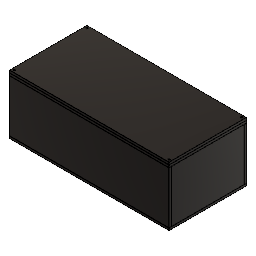
Battery Box ABS Panel v19 (Autodesk Fusion 360 design; units mm, degrees)
Autodesk Fusion 360 part; units mm, degrees
sketch "Sketch1" plane through (0, 0, 0) normal (0, 1, 0) x (1, 0, 0)
  line L0 (197.5, -96) -> (-197.5, -96)
  line L1 (-197.5, -96) -> (-197.5, 96)
  line L2 (-197.5, 96) -> (197.5, 96)
  line L3 (197.5, 96) -> (197.5, -96)
  line L4 (197.5, -96) -> (-197.5, 96) construction
  line L5 (-197.5, -96) -> (197.5, 96) construction
  line L6 (-197.5, 0) -> (197.5, 0) construction
  line L7 (0, 96) -> (0, -96) construction
  dimension "loa" = 395
  dimension "woa" = 192
  constraint horizontal L0
  constraint perpendicular L0 L1
  constraint parallel L0 L2
  constraint parallel L1 L3
  constraint coincident L4 origin
  constraint coincident L5 origin
  constraint midpoint L1 L6.start
  constraint midpoint L3 L6.end
  constraint midpoint L2 L7.start
  constraint midpoint L0 L7.end
  measures "loa" distance of L1.end L2.end
  measures "woa" distance of L0.end L1.end
extrude "Extrude1" add sketch "Sketch1" along normal blind 6 makes body 1
sketch "Sketch9" plane through (0, 6, 0) normal (0, 1, 0) x (-1, 0, 0)
  line L0 (-197.5, -96) -> (197.5, -96)
  line L1 (197.5, -96) -> (197.5, 96)
  line L2 (-197.5, 96) -> (-197.5, -96)
  circle A0 centre (191.5, -90) radius 3
  line L3 (195.85, -71) -> (195.85, -74.7217)
  arc A1 (190.1785, -83.3177) -> (195.85, -74.7217) centre (186.5, -74.7217) ccw
  line L4 (190.1785, -83.3177) -> (187.9545, -84.2694)
  arc A2 (187.9545, -84.2694) -> (185.4753, -86.7956) centre (189.7839, -88.5444) ccw
  line L5 (184.7768, -88.5165) -> (185.4753, -86.7956)
  arc A3 (176.1133, -94.35) -> (184.7768, -88.5165) centre (176.1133, -85) ccw
  line L6 (172.5, -94.35) -> (176.1133, -94.35)
  line L7 (172.5, -91.65) -> (176.1133, -91.65)
  arc A4 (176.1133, -91.65) -> (182.275, -87.501) centre (176.1133, -85) ccw
  line L8 (182.275, -87.501) -> (182.9735, -85.7802)
  arc A5 (186.8923, -81.7871) -> (182.9735, -85.7802) centre (189.7839, -88.5444) ccw
  line L9 (189.1162, -80.8354) -> (186.8923, -81.7871)
  arc A6 (189.1162, -80.8354) -> (193.15, -74.7217) centre (186.5, -74.7217) ccw
  line L10 (193.15, -71) -> (193.15, -74.7217)
  line L11 (197.5, 0.1916) -> (197.5, -96)
  line L12 (197.5, -96) -> (0, -96)
  line L13 (193.15, -71) -> (193.0809, 0.1873)
  line L14 (195.85, -71) -> (195.7809, 0.1899)
  line L15 (172.5, -94.35) -> (0, -94.35)
  line L16 (172.5, -91.65) -> (0, -91.65)
  line L17 (172.5, -90) -> (0, -90)
  line L18 (172.5, -90) -> (176.1133, -90)
  arc A7 (176.1133, -90) -> (180.7462, -86.8805) centre (176.1133, -85) ccw
  line L19 (180.7462, -86.8805) -> (181.4446, -85.1596)
  arc A8 (186.2431, -80.2702) -> (181.4446, -85.1596) centre (189.7839, -88.5444) ccw
  line L20 (188.4671, -79.3185) -> (186.2431, -80.2702)
  arc A9 (188.4671, -79.3185) -> (191.5, -74.7217) centre (186.5, -74.7217) ccw
  line L21 (191.5, -71.0008) -> (191.5, -74.7217)
  line L22 (191.5, -71.0008) -> (191.4309, 0.1857)
  line L23 (197.5, 0.1916) -> (191.4309, 0.1857)
  line L24 (0, -96) -> (0, -90)
  point P0 (191.5, -80.0006)
  point P1 (181.5, -80.0006)
  point P2 (181.5, -90.0006)
  point P3 (194.5, -80)
  point P4 (181.5, -93)
  dimension "d74" = 10
  dimension "d75" = 10
  dimension "d80" = 6
  dimension "d97" = 6
  dimension "d98" = 6
  dimension "d99" = -1.65
  constraint coincident L0.end L1.start
  constraint tangent L5 A3
  constraint tangent L4 A2
  constraint tangent A3 L6
  constraint tangent L3 A1
  constraint tangent A2 L5
  constraint tangent A1 L4
  constraint tangent A6 L10
  constraint tangent L9 A6
  constraint tangent A5 L9
  constraint tangent A4 L8
  constraint tangent L7 A4
  constraint tangent L8 A5
  constraint vertical L11
  constraint horizontal L12
  constraint perpendicular L22 L23
  constraint perpendicular L17 L24
  measures "d74" distance of P0 P1
  measures "d75" distance of P1 P2
  measures "d80" diameter of A0
  measures "d97" distance of A0.centre L12
  measures "d98" distance of A0.centre L11
sketch "Sketch2" plane through (0, 6, 0) normal (0, 1, 0) x (-1, 0, 0)
  line L0 (-181, 79.5) -> (181, 79.5)
  line L1 (181, 79.5) -> (181, -79.5)
  line L2 (181, -79.5) -> (-181, -79.5)
  line L3 (-181, -79.5) -> (-181, 79.5)
  line L4 (-181, 79.5) -> (181, -79.5) construction
  line L5 (181, 79.5) -> (-181, -79.5) construction
  line L6 (183, 81.5) -> (183, -81.5)
  line L7 (183, -81.5) -> (-183, -81.5)
  line L8 (-183, -81.5) -> (-183, 81.5)
  line L9 (-183, 81.5) -> (183, 81.5)
  line L10 (-197.5, -96) -> (197.5, -96)
  line L11 (197.5, -96) -> (197.5, 96)
  line L12 (197.5, 96) -> (-197.5, 96)
  line L13 (-197.5, 96) -> (-197.5, -96)
  dimension "d14" = 159
  dimension "d15" = 362
  dimension "d16" = -2
  constraint horizontal L0
  constraint perpendicular L0 L1
  constraint parallel L0 L2
  constraint parallel L1 L3
  constraint coincident L4 origin
  constraint coincident L5 origin
  measures "d14" distance of L0.end L1.end
  measures "d15" distance of L1.end L2.end
sketch "Sketch3" plane through (0, 6, 0) normal (0, 1, 0) x (-1, 0, 0)
  line L0 (-180, 78.5) -> (180, 78.5)
  line L1 (180, 78.5) -> (180, -78.5)
  line L2 (180, -78.5) -> (-180, -78.5)
  line L3 (-180, -78.5) -> (-180, 78.5)
  line L4 (-180, 78.5) -> (180, -78.5) construction
  line L5 (180, 78.5) -> (-180, -78.5) construction
  line L6 (-197.5, -96) -> (197.5, -96)
  line L7 (197.5, -96) -> (197.5, 96)
  line L8 (197.5, 96) -> (-197.5, 96)
  line L9 (-197.5, 96) -> (-197.5, -96)
  dimension "d19" = 360
  dimension "d20" = 157
  constraint horizontal L0
  constraint perpendicular L0 L1
  constraint parallel L0 L2
  constraint parallel L1 L3
  constraint coincident L4 origin
  constraint coincident L5 origin
  measures "d19" distance of L1.end L2.end
  measures "d20" distance of L0.end L1.end
extrude "Extrude4" add sketch "Sketch3" along normal blind 80 separate body contours L0 L1 L2 L3 makes body 2
sketch "Sketch4" plane through (0, 86, 0) normal (0, 1, 0) x (-1, 0, 0)
  line L0 (-180, -78.5) -> (180, -78.5)
  line L1 (180, -78.5) -> (180, 78.5)
  line L2 (180, 78.5) -> (-180, 78.5)
  line L3 (-180, 78.5) -> (-180, -78.5)
  line L4 (-42.5, 65) -> (42.5, 65)
  line L5 (42.5, 65) -> (42.5, -65)
  line L6 (42.5, -65) -> (-42.5, -65)
  line L7 (-42.5, -65) -> (-42.5, 65)
  line L8 (-42.5, 65) -> (42.5, -65) construction
  line L9 (42.5, 65) -> (-42.5, -65) construction
  dimension "d23" = 85
  dimension "d24" = 130
  constraint horizontal L4
  constraint perpendicular L4 L5
  constraint parallel L4 L6
  constraint parallel L5 L7
  constraint coincident L8 origin
  constraint coincident L9 origin
  measures "d23" distance of L5.end L6.end
  measures "d24" distance of L4.end L5.end
extrude "Extrude5" add sketch "Sketch4" along normal blind 36 separate body contours L4 L5 L6 L7 makes body 3
box "BoxPrimitive1" add length 6 width 395 height 129 placed x (0, 0, 1) y (1, 0, 0) z (0, 1, 0) at (-197.5, 6, -96) separate body makes body 4
mirror "Mirror3" about plane through (0, 0, 0) normal (0, 0, 1) of bodies 4 makes body 5
sketch "Sketch14" plane through (0, 6, 0) normal (0, 1, 0) x (-1, 0, 0)
  line L0 (-197.5, -96) -> (197.5, -96)
  line L1 (197.5, -96) -> (197.5, 96)
  line L2 (197.5, 96) -> (-197.5, 96)
  line L3 (-197.5, 96) -> (-197.5, -96)
  line L4 (197.5, 90) -> (-197.5, 90)
  line L5 (-197.5, -90) -> (197.5, -90)
  line L6 (197.5, 90) -> (191.5, 90)
  line L7 (191.5, 90) -> (191.5, -90)
  line L8 (191.5, -90) -> (197.5, -90)
  line L9 (197.5, -90) -> (197.5, 90)
  dimension "d118" = 6
  constraint horizontal L6
  constraint vertical L7
  constraint horizontal L8
  constraint vertical L9
  constraint coincident L4.start L6.start
  measures "d118" distance of L4.start L6.end
extrude "Extrude13" add sketch "Sketch14" along normal blind 129 separate body contours L1 L4 L5 L6 L7 L8 L9 makes body 6
mirror "Mirror4" about plane through (0, 0, 0) normal (1, 0, 0) of bodies 6 makes body 7
sketch "Sketch16" plane through (0, 135, 0) normal (0, 1, 0) x (-1, 0, 0)
  line L0 (197.5, -90) -> (-197.5, -90)
  line L1 (-197.5, -90) -> (-197.5, -96)
  line L2 (-197.5, -96) -> (197.5, -96)
  line L3 (197.5, -96) -> (197.5, -90)
  line L4 (197.5, -96) -> (0, -96)
  line L5 (197.5, 0.1916) -> (197.5, -96)
  line L6 (191.5, -71.0008) -> (191.4309, 0.1857)
  line L7 (172.5, -94.35) -> (0, -94.35)
  line L8 (172.5, -91.65) -> (0, -91.65)
  line L9 (172.5, -90) -> (0, -90)
  line L10 (172.5, -94.35) -> (176.1133, -94.35)
  arc A0 (176.1133, -94.35) -> (184.7768, -88.5165) centre (176.1133, -85) ccw
  circle A1 centre (191.5, -90) radius 3
  line L11 (184.7768, -88.5165) -> (185.4753, -86.7956)
  arc A2 (187.9545, -84.2694) -> (185.4753, -86.7956) centre (189.7839, -88.5444) ccw
  line L12 (190.1785, -83.3177) -> (187.9545, -84.2694)
  arc A3 (190.1785, -83.3177) -> (195.85, -74.7217) centre (186.5, -74.7217) ccw
  line L13 (195.85, -71) -> (195.85, -74.7217)
  line L14 (195.85, -71) -> (195.7809, 0.1899)
  line L15 (193.15, -71) -> (193.0809, 0.1873)
  line L16 (193.15, -71) -> (193.15, -74.7217)
  line L17 (191.5, -71.0008) -> (191.5, -74.7217)
  arc A4 (189.1162, -80.8354) -> (193.15, -74.7217) centre (186.5, -74.7217) ccw
  line L18 (189.1162, -80.8354) -> (186.8923, -81.7871)
  arc A5 (188.4671, -79.3185) -> (191.5, -74.7217) centre (186.5, -74.7217) ccw
  line L19 (188.4671, -79.3185) -> (186.2431, -80.2702)
  arc A6 (186.2431, -80.2702) -> (181.4446, -85.1596) centre (189.7839, -88.5444) ccw
  arc A7 (186.8923, -81.7871) -> (182.9735, -85.7802) centre (189.7839, -88.5444) ccw
  line L20 (182.275, -87.501) -> (182.9735, -85.7802)
  line L21 (180.7462, -86.8805) -> (181.4446, -85.1596)
  arc A8 (176.1133, -91.65) -> (182.275, -87.501) centre (176.1133, -85) ccw
  line L22 (172.5, -91.65) -> (176.1133, -91.65)
  line L23 (172.5, -90) -> (176.1133, -90)
  arc A9 (176.1133, -90) -> (180.7462, -86.8805) centre (176.1133, -85) ccw
  line L24 (197.5, 0.1916) -> (191.4309, 0.1857)
  line L25 (0, -96) -> (0, -90)
  constraint coincident L5.start L24.start
  constraint coincident L6.end L24.end
  constraint coincident L4.end L25.start
  constraint coincident L9.end L25.end
extrude "Extrude14" add sketch "Sketch16" along normal blind 6 separate body contours L0 L2 L3 L4 L5 L7 L10 A0 A1 L25 | L0 L5 A0 A1 L11 A2 L12 A3 L13 L14 L24 | L0 A0 L11 A2 L12 A3 L13 L14 L15 L16 A4 L18 A7 L20 A8 L24 | L0 L7 L8 L10 A0 A8 L22 L25 | L0 L6 L15 L16 L17 A4 L18 A5 L19 A6 A7 L20 L21 A8 A9 L24 | L0 L8 L9 A8 L22 L23 L25 makes body 8
sketch "Sketch17" plane through (0, 141, 0) normal (0, 1, 0) x (-1, 0, 0)
  circle A0 centre (191.5, -90) radius 3
  line L0 (197.5, 0.1916) -> (191.4309, 0.1857)
  line L1 (191.4309, 0.1857) -> (191.5, -71.0008)
  line L2 (191.5, -71.0008) -> (191.5, -74.7217)
  arc A1 (188.4671, -79.3185) -> (191.5, -74.7217) centre (186.5, -74.7217) ccw
  line L3 (188.4671, -79.3185) -> (186.2431, -80.2702)
  arc A2 (186.2431, -80.2702) -> (181.4446, -85.1596) centre (189.7839, -88.5444) ccw
  line L4 (181.4446, -85.1596) -> (180.7462, -86.8805)
  arc A3 (176.1133, -90) -> (180.7462, -86.8805) centre (176.1133, -85) ccw
  line L5 (176.1133, -90) -> (172.5, -90)
  line L6 (172.5, -90) -> (0, -90)
  line L7 (0, -90) -> (0, -96)
  line L8 (0, -96) -> (197.5, -96)
  line L9 (197.5, -96) -> (197.5, 0.1916)
  line L10 (195.85, -71) -> (195.7809, 0.1899)
  line L11 (193.15, -71) -> (193.0809, 0.1873)
  line L12 (195.85, -71) -> (195.85, -74.7217)
  line L13 (193.15, -71) -> (193.15, -74.7217)
  arc A4 (190.1785, -83.3177) -> (195.85, -74.7217) centre (186.5, -74.7217) ccw
  arc A5 (189.1162, -80.8354) -> (193.15, -74.7217) centre (186.5, -74.7217) ccw
  line L14 (190.1785, -83.3177) -> (187.9545, -84.2694)
  arc A6 (187.9545, -84.2694) -> (185.4753, -86.7956) centre (189.7839, -88.5444) ccw
  line L15 (189.1162, -80.8354) -> (186.8923, -81.7871)
  arc A7 (186.8923, -81.7871) -> (182.9735, -85.7802) centre (189.7839, -88.5444) ccw
  line L16 (182.275, -87.501) -> (182.9735, -85.7802)
  arc A8 (176.1133, -91.65) -> (182.275, -87.501) centre (176.1133, -85) ccw
  line L17 (184.7768, -88.5165) -> (185.4753, -86.7956)
  arc A9 (176.1133, -94.35) -> (184.7768, -88.5165) centre (176.1133, -85) ccw
  line L18 (172.5, -94.35) -> (176.1133, -94.35)
  line L19 (172.5, -91.65) -> (176.1133, -91.65)
  line L20 (172.5, -94.35) -> (0, -94.35)
  line L21 (172.5, -91.65) -> (0, -91.65)
extrude "Extrude15" cut sketch "Sketch17" against normal blind 1.35 contours L0 L7 L10 L11 L12 L13 A4 A5 L14 A6 L15 A7 L16 A8 L17 A9 L18 L19 L20 L21 bodies 8
sketch "Export Side" plane through (197.5, 0, 0) normal (1, 0, 0) x (0, 0, -1)
  line L0 (-90, 6) -> (90, 6)
  line L1 (90, 6) -> (90, 135)
  line L2 (90, 135) -> (-90, 135)
  line L3 (-90, 135) -> (-90, 6)
sketch "Export Side Long" plane through (0, 0, 96) normal (0, 0, 1) x (1, 0, 0)
  line L0 (197.5, 6) -> (197.5, 135)
  line L1 (197.5, 135) -> (-197.5, 135)
  line L2 (-197.5, 135) -> (-197.5, 6)
  line L3 (-197.5, 6) -> (197.5, 6)
mirror "Mirror5" about plane through (0, 0, 0) normal (0, 0, 1) of bodies 8 merged
mirror "Mirror6" about plane through (0, 0, 0) normal (1, 0, 0) of bodies 8 merged
box "BoxPrimitive3" add length 192 width 395 height 6 placed x (0, 0, 1) y (1, 0, 0) z (0, 1, 0) at (-197.5, 141, -96) separate body makes body 9
sketch "Sketch21" plane through (0, 147, 0) normal (0, 1, 0) x (-1, 0, 0)
  line L0 (197.5, 96) -> (-197.5, 96)
  line L1 (-197.5, 96) -> (-197.5, -96)
  line L2 (-197.5, -96) -> (197.5, -96)
  line L3 (197.5, -96) -> (197.5, 96)
  circle A0 centre (191.5, -90) radius 3
  circle A1 centre (-191.5, -90) radius 3
  circle A2 centre (-191.5, 90) radius 3
  circle A3 centre (191.5, 90) radius 3
  point P0 (191.5, -90)
hole "Hole1" at (-191.5, 147, -90) at (191.5, 147, -90) at (191.5, 147, 90) at (-191.5, 147, 90) direction (0, -1, 0) diameter 4.2 depth 6 tip angle 118 bodies 9
sketch "Export Lid" plane through (0, 147, 0) normal (0, 1, 0) x (-1, 0, 0)
  circle A0 centre (-191.5, 90) radius 2.1
  circle A1 centre (191.5, -90) radius 2.1
  circle A2 centre (-191.5, -90) radius 2.1
  circle A3 centre (191.5, 90) radius 2.1
  line L0 (197.5, 96) -> (-197.5, 96)
  line L1 (-197.5, 96) -> (-197.5, -96)
  line L2 (-197.5, -96) -> (197.5, -96)
  line L3 (197.5, -96) -> (197.5, 96)
sketch "Export Lip" plane through (0, 141, 0) normal (0, 1, 0) x (-1, 0, 0)
  line L0 (0, 94.35) -> (172.5, 94.35)
  line L1 (172.5, 94.35) -> (176.1133, 94.35)
  arc A0 (184.7768, 88.5165) -> (176.1133, 94.35) centre (176.1133, 85) ccw
  line L2 (184.7768, 88.5165) -> (185.4753, 86.7956)
  arc A1 (185.4753, 86.7956) -> (187.9545, 84.2694) centre (189.7839, 88.5444) ccw
  line L3 (187.9545, 84.2694) -> (190.1785, 83.3177)
  arc A2 (195.85, 74.7217) -> (190.1785, 83.3177) centre (186.5, 74.7217) ccw
  line L4 (195.85, 74.7217) -> (195.85, 71)
  line L5 (195.85, 71) -> (195.7813, 0.1899)
  line L6 (195.7813, 0.1899) -> (195.7809, 0.1899)
  line L7 (195.7809, 0.1899) -> (195.7811, 0)
  line L8 (195.7811, 0) -> (195.7809, -0.1899)
  line L9 (195.7809, -0.1899) -> (195.7813, -0.1899)
  line L10 (195.7813, -0.1899) -> (195.85, -71)
  line L11 (195.85, -71) -> (195.85, -74.7217)
  arc A3 (190.1785, -83.3177) -> (195.85, -74.7217) centre (186.5, -74.7217) ccw
  line L12 (190.1785, -83.3177) -> (187.9545, -84.2694)
  arc A4 (187.9545, -84.2694) -> (185.4753, -86.7956) centre (189.7839, -88.5444) ccw
  line L13 (185.4753, -86.7956) -> (184.7768, -88.5165)
  arc A5 (176.1133, -94.35) -> (184.7768, -88.5165) centre (176.1133, -85) ccw
  line L14 (176.1133, -94.35) -> (172.5, -94.35)
  line L15 (172.5, -94.35) -> (0, -94.35)
  line L16 (0, -94.35) -> (-172.5, -94.35)
  line L17 (-172.5, -94.35) -> (-176.1133, -94.35)
  arc A6 (-184.7768, -88.5165) -> (-176.1133, -94.35) centre (-176.1133, -85) ccw
  line L18 (-184.7768, -88.5165) -> (-185.4753, -86.7956)
  arc A7 (-185.4753, -86.7956) -> (-187.9545, -84.2694) centre (-189.7839, -88.5444) ccw
  line L19 (-187.9545, -84.2694) -> (-190.1785, -83.3177)
  arc A8 (-195.85, -74.7217) -> (-190.1785, -83.3177) centre (-186.5, -74.7217) ccw
  line L20 (-195.85, -74.7217) -> (-195.85, -71)
  line L21 (-195.85, -71) -> (-195.7813, -0.1899)
  line L22 (-195.7813, -0.1899) -> (-195.7809, -0.1899)
  line L23 (-195.7809, -0.1899) -> (-195.7811, 0)
  line L24 (-195.7811, 0) -> (-195.7809, 0.1899)
  line L25 (-195.7809, 0.1899) -> (-195.7813, 0.1899)
  line L26 (-195.7813, 0.1899) -> (-195.85, 71)
  line L27 (-195.85, 71) -> (-195.85, 74.7217)
  arc A9 (-190.1785, 83.3177) -> (-195.85, 74.7217) centre (-186.5, 74.7217) ccw
  line L28 (-190.1785, 83.3177) -> (-187.9545, 84.2694)
  arc A10 (-187.9545, 84.2694) -> (-185.4753, 86.7956) centre (-189.7839, 88.5444) ccw
  line L29 (-185.4753, 86.7956) -> (-184.7768, 88.5165)
  arc A11 (-176.1133, 94.35) -> (-184.7768, 88.5165) centre (-176.1133, 85) ccw
  line L30 (-176.1133, 94.35) -> (-172.5, 94.35)
  line L31 (-172.5, 94.35) -> (0, 94.35)
  circle A12 centre (-191.5, -90) radius 3
  circle A13 centre (-191.5, 90) radius 3
  circle A14 centre (191.5, 90) radius 3
  circle A15 centre (191.5, -90) radius 3
  line L32 (0, 96) -> (-197.5, 96)
  line L33 (-197.5, 96) -> (-197.5, -96)
  line L34 (-197.5, -96) -> (0, -96)
  line L35 (0, -96) -> (197.5, -96)
  line L36 (197.5, -96) -> (197.5, 96)
  line L37 (197.5, 96) -> (0, 96)
  line L38 (0, 90) -> (172.5, 90)
  line L39 (172.5, 90) -> (176.1133, 90)
  arc A16 (180.7462, 86.8805) -> (176.1133, 90) centre (176.1133, 85) ccw
  line L40 (180.7462, 86.8805) -> (181.4446, 85.1596)
  arc A17 (181.4446, 85.1596) -> (186.2431, 80.2702) centre (189.7839, 88.5444) ccw
  line L41 (186.2431, 80.2702) -> (188.4671, 79.3185)
  arc A18 (191.5, 74.7217) -> (188.4671, 79.3185) centre (186.5, 74.7217) ccw
  line L42 (191.5, 74.7217) -> (191.5, 71.0008)
  line L43 (191.5, 71.0008) -> (191.4313, 0.1857)
  line L44 (191.4313, 0.1857) -> (191.4309, 0.1857)
  line L45 (191.4309, 0.1857) -> (191.4311, 0)
  line L46 (191.4311, 0) -> (191.4309, -0.1857)
  line L47 (191.4309, -0.1857) -> (191.4313, -0.1857)
  line L48 (191.4313, -0.1857) -> (191.5, -71.0008)
  line L49 (191.5, -71.0008) -> (191.5, -74.7217)
  arc A19 (188.4671, -79.3185) -> (191.5, -74.7217) centre (186.5, -74.7217) ccw
  line L50 (188.4671, -79.3185) -> (186.2431, -80.2702)
  arc A20 (186.2431, -80.2702) -> (181.4446, -85.1596) centre (189.7839, -88.5444) ccw
  line L51 (181.4446, -85.1596) -> (180.7462, -86.8805)
  arc A21 (176.1133, -90) -> (180.7462, -86.8805) centre (176.1133, -85) ccw
  line L52 (176.1133, -90) -> (172.5, -90)
  line L53 (172.5, -90) -> (0, -90)
  line L54 (0, -90) -> (-172.5, -90)
  line L55 (-172.5, -90) -> (-176.1133, -90)
  arc A22 (-180.7462, -86.8805) -> (-176.1133, -90) centre (-176.1133, -85) ccw
  line L56 (-180.7462, -86.8805) -> (-181.4446, -85.1596)
  arc A23 (-181.4446, -85.1596) -> (-186.2431, -80.2702) centre (-189.7839, -88.5444) ccw
  line L57 (-186.2431, -80.2702) -> (-188.4671, -79.3185)
  arc A24 (-191.5, -74.7217) -> (-188.4671, -79.3185) centre (-186.5, -74.7217) ccw
  line L58 (-191.5, -74.7217) -> (-191.5, -71.0008)
  line L59 (-191.5, -71.0008) -> (-191.4313, -0.1857)
  line L60 (-191.4313, -0.1857) -> (-191.4309, -0.1857)
  line L61 (-191.4309, -0.1857) -> (-191.4311, 0)
  line L62 (-191.4311, 0) -> (-191.4309, 0.1857)
  line L63 (-191.4309, 0.1857) -> (-191.4313, 0.1857)
  line L64 (-191.4313, 0.1857) -> (-191.5, 71.0008)
  line L65 (-191.5, 71.0008) -> (-191.5, 74.7217)
  arc A25 (-188.4671, 79.3185) -> (-191.5, 74.7217) centre (-186.5, 74.7217) ccw
  line L66 (-188.4671, 79.3185) -> (-186.2431, 80.2702)
  arc A26 (-186.2431, 80.2702) -> (-181.4446, 85.1596) centre (-189.7839, 88.5444) ccw
  line L67 (-181.4446, 85.1596) -> (-180.7462, 86.8805)
  arc A27 (-176.1133, 90) -> (-180.7462, 86.8805) centre (-176.1133, 85) ccw
  line L68 (-176.1133, 90) -> (-172.5, 90)
  line L69 (-172.5, 90) -> (0, 90)
  line L70 (0, 91.65) -> (-172.5, 91.65)
  line L71 (-172.5, 91.65) -> (-176.1133, 91.65)
  arc A28 (-176.1133, 91.65) -> (-182.275, 87.501) centre (-176.1133, 85) ccw
  line L72 (-182.275, 87.501) -> (-182.9735, 85.7802)
  arc A29 (-186.8923, 81.7871) -> (-182.9735, 85.7802) centre (-189.7839, 88.5444) ccw
  line L73 (-186.8923, 81.7871) -> (-189.1162, 80.8354)
  arc A30 (-189.1162, 80.8354) -> (-193.15, 74.7217) centre (-186.5, 74.7217) ccw
  line L74 (-193.15, 74.7217) -> (-193.15, 71)
  line L75 (-193.15, 71) -> (-193.0811, 0)
  line L76 (-193.0811, 0) -> (-193.15, -71)
  line L77 (-193.15, -71) -> (-193.15, -74.7217)
  arc A31 (-193.15, -74.7217) -> (-189.1162, -80.8354) centre (-186.5, -74.7217) ccw
  line L78 (-189.1162, -80.8354) -> (-186.8923, -81.7871)
  arc A32 (-182.9735, -85.7802) -> (-186.8923, -81.7871) centre (-189.7839, -88.5444) ccw
  line L79 (-182.9735, -85.7802) -> (-182.275, -87.501)
  arc A33 (-182.275, -87.501) -> (-176.1133, -91.65) centre (-176.1133, -85) ccw
  line L80 (-176.1133, -91.65) -> (-172.5, -91.65)
  line L81 (-172.5, -91.65) -> (0, -91.65)
  line L82 (0, -91.65) -> (172.5, -91.65)
  line L83 (172.5, -91.65) -> (176.1133, -91.65)
  arc A34 (176.1133, -91.65) -> (182.275, -87.501) centre (176.1133, -85) ccw
  line L84 (182.275, -87.501) -> (182.9735, -85.7802)
  arc A35 (186.8923, -81.7871) -> (182.9735, -85.7802) centre (189.7839, -88.5444) ccw
  line L85 (186.8923, -81.7871) -> (189.1162, -80.8354)
  arc A36 (189.1162, -80.8354) -> (193.15, -74.7217) centre (186.5, -74.7217) ccw
  line L86 (193.15, -74.7217) -> (193.15, -71)
  line L87 (193.15, -71) -> (193.0811, 0)
  line L88 (193.0811, 0) -> (193.15, 71)
  line L89 (193.15, 71) -> (193.15, 74.7217)
  arc A37 (193.15, 74.7217) -> (189.1162, 80.8354) centre (186.5, 74.7217) ccw
  line L90 (189.1162, 80.8354) -> (186.8923, 81.7871)
  arc A38 (182.9735, 85.7802) -> (186.8923, 81.7871) centre (189.7839, 88.5444) ccw
  line L91 (182.9735, 85.7802) -> (182.275, 87.501)
  arc A39 (182.275, 87.501) -> (176.1133, 91.65) centre (176.1133, 85) ccw
  line L92 (176.1133, 91.65) -> (172.5, 91.65)
  line L93 (172.5, 91.65) -> (0, 91.65)
  line L94 (0, 91.65) -> (172.5, 91.65)
  line L95 (172.5, 91.65) -> (176.1133, 91.65)
  arc A40 (182.275, 87.501) -> (176.1133, 91.65) centre (176.1133, 85) ccw
  line L96 (182.275, 87.501) -> (182.9735, 85.7802)
  arc A41 (182.9735, 85.7802) -> (186.8923, 81.7871) centre (189.7839, 88.5444) ccw
  line L97 (186.8923, 81.7871) -> (189.1162, 80.8354)
  arc A42 (193.15, 74.7217) -> (189.1162, 80.8354) centre (186.5, 74.7217) ccw
  line L98 (193.15, 74.7217) -> (193.15, 71)
  line L99 (193.15, 71) -> (193.0811, 0)
  line L100 (193.0811, 0) -> (193.15, -71)
  line L101 (193.15, -71) -> (193.15, -74.7217)
  arc A43 (189.1162, -80.8354) -> (193.15, -74.7217) centre (186.5, -74.7217) ccw
  line L102 (189.1162, -80.8354) -> (186.8923, -81.7871)
  arc A44 (186.8923, -81.7871) -> (182.9735, -85.7802) centre (189.7839, -88.5444) ccw
  line L103 (182.9735, -85.7802) -> (182.275, -87.501)
  arc A45 (176.1133, -91.65) -> (182.275, -87.501) centre (176.1133, -85) ccw
  line L104 (176.1133, -91.65) -> (172.5, -91.65)
  line L105 (172.5, -91.65) -> (0, -91.65)
  line L106 (0, -91.65) -> (-172.5, -91.65)
  line L107 (-172.5, -91.65) -> (-176.1133, -91.65)
  arc A46 (-182.275, -87.501) -> (-176.1133, -91.65) centre (-176.1133, -85) ccw
  line L108 (-182.275, -87.501) -> (-182.9735, -85.7802)
  arc A47 (-182.9735, -85.7802) -> (-186.8923, -81.7871) centre (-189.7839, -88.5444) ccw
  line L109 (-186.8923, -81.7871) -> (-189.1162, -80.8354)
  arc A48 (-193.15, -74.7217) -> (-189.1162, -80.8354) centre (-186.5, -74.7217) ccw
  line L110 (-193.15, -74.7217) -> (-193.15, -71)
  line L111 (-193.15, -71) -> (-193.0811, 0)
  line L112 (-193.0811, 0) -> (-193.15, 71)
  line L113 (-193.15, 71) -> (-193.15, 74.7217)
  arc A49 (-189.1162, 80.8354) -> (-193.15, 74.7217) centre (-186.5, 74.7217) ccw
  line L114 (-189.1162, 80.8354) -> (-186.8923, 81.7871)
  arc A50 (-186.8923, 81.7871) -> (-182.9735, 85.7802) centre (-189.7839, 88.5444) ccw
  line L115 (-182.9735, 85.7802) -> (-182.275, 87.501)
  arc A51 (-176.1133, 91.65) -> (-182.275, 87.501) centre (-176.1133, 85) ccw
  line L116 (-176.1133, 91.65) -> (-172.5, 91.65)
  line L117 (-172.5, 91.65) -> (0, 91.65)
  line L118 (0, 94.35) -> (-172.5, 94.35)
  line L119 (-172.5, 94.35) -> (-176.1133, 94.35)
  arc A52 (-176.1133, 94.35) -> (-184.7768, 88.5165) centre (-176.1133, 85) ccw
  line L120 (-184.7768, 88.5165) -> (-185.4753, 86.7956)
  arc A53 (-187.9545, 84.2694) -> (-185.4753, 86.7956) centre (-189.7839, 88.5444) ccw
  line L121 (-187.9545, 84.2694) -> (-190.1785, 83.3177)
  arc A54 (-190.1785, 83.3177) -> (-195.85, 74.7217) centre (-186.5, 74.7217) ccw
  line L122 (-195.85, 74.7217) -> (-195.85, 71)
  line L123 (-195.85, 71) -> (-195.7813, 0.1899)
  line L124 (-195.7813, 0.1899) -> (-195.7809, 0.1899)
  line L125 (-195.7809, 0.1899) -> (-195.7811, 0)
  line L126 (-195.7811, 0) -> (-195.7809, -0.1899)
  line L127 (-195.7809, -0.1899) -> (-195.7813, -0.1899)
  line L128 (-195.7813, -0.1899) -> (-195.85, -71)
  line L129 (-195.85, -71) -> (-195.85, -74.7217)
  arc A55 (-195.85, -74.7217) -> (-190.1785, -83.3177) centre (-186.5, -74.7217) ccw
  line L130 (-190.1785, -83.3177) -> (-187.9545, -84.2694)
  arc A56 (-185.4753, -86.7956) -> (-187.9545, -84.2694) centre (-189.7839, -88.5444) ccw
  line L131 (-185.4753, -86.7956) -> (-184.7768, -88.5165)
  arc A57 (-184.7768, -88.5165) -> (-176.1133, -94.35) centre (-176.1133, -85) ccw
  line L132 (-176.1133, -94.35) -> (-172.5, -94.35)
  line L133 (-172.5, -94.35) -> (0, -94.35)
  line L134 (0, -94.35) -> (172.5, -94.35)
  line L135 (172.5, -94.35) -> (176.1133, -94.35)
  arc A58 (176.1133, -94.35) -> (184.7768, -88.5165) centre (176.1133, -85) ccw
  line L136 (184.7768, -88.5165) -> (185.4753, -86.7956)
  arc A59 (187.9545, -84.2694) -> (185.4753, -86.7956) centre (189.7839, -88.5444) ccw
  line L137 (187.9545, -84.2694) -> (190.1785, -83.3177)
  arc A60 (190.1785, -83.3177) -> (195.85, -74.7217) centre (186.5, -74.7217) ccw
  line L138 (195.85, -74.7217) -> (195.85, -71)
  line L139 (195.85, -71) -> (195.7813, -0.1899)
  line L140 (195.7813, -0.1899) -> (195.7809, -0.1899)
  line L141 (195.7809, -0.1899) -> (195.7811, 0)
  line L142 (195.7811, 0) -> (195.7809, 0.1899)
  line L143 (195.7809, 0.1899) -> (195.7813, 0.1899)
  line L144 (195.7813, 0.1899) -> (195.85, 71)
  line L145 (195.85, 71) -> (195.85, 74.7217)
  arc A61 (195.85, 74.7217) -> (190.1785, 83.3177) centre (186.5, 74.7217) ccw
  line L146 (190.1785, 83.3177) -> (187.9545, 84.2694)
  arc A62 (185.4753, 86.7956) -> (187.9545, 84.2694) centre (189.7839, 88.5444) ccw
  line L147 (185.4753, 86.7956) -> (184.7768, 88.5165)
  arc A63 (184.7768, 88.5165) -> (176.1133, 94.35) centre (176.1133, 85) ccw
  line L148 (176.1133, 94.35) -> (172.5, 94.35)
  line L149 (172.5, 94.35) -> (0, 94.35)
sketch "Sketch24" plane through (0, 0, -96) normal (0, 0, -1) x (-1, 0, 0)
  line L0 (-197.5, 135) -> (-197.5, 6)
  line L1 (-197.5, 6) -> (197.5, 6)
  line L2 (197.5, 6) -> (197.5, 135)
  line L3 (197.5, 135) -> (-197.5, 135)
  circle A0 centre (-160, 113) radius 13.5
  line L4 (0, 1.75) -> (0, 22.5)
  circle A1 centre (160, 113) radius 13.5
  dimension "d144" = 27
  dimension "d146" = 22
  constraint symmetric A0 L4 A1
  measures "d144" diameter of A0
  measures "d146" distance of L3 A0.centre
extrude "Extrude16" cut sketch "Sketch24" against normal through all contours A0 | A1 bodies 4
sketch "Export Back" plane through (0, 0, -96) normal (0, 0, -1) x (-1, 0, 0)
  circle A0 centre (160, 113) radius 13.5
  circle A1 centre (-160, 113) radius 13.5
  line L0 (-197.5, 135) -> (-197.5, 6)
  line L1 (-197.5, 6) -> (197.5, 6)
  line L2 (197.5, 6) -> (197.5, 135)
  line L3 (197.5, 135) -> (-197.5, 135)
copy_body "Body->Comp1" bodies 2 removing the originals makes body 10 in component "Battery"
copy_body "Body->Comp2" bodies 3 removing the originals makes body 11 in component "Controller"
component "Battery" placed x (1, 0, 0) y (0, 1, 0) z (0, 0, 1) at (0, 0, 0)
component "Controller" placed x (1, 0, 0) y (0, 1, 0) z (0, 0, 1) at (0, 0, 0)
equation "corner = 16 mm"
equation "wallThickness = 6 mm"
equation "d7 = wallThickness"
equation "hoa = 135 mm"
equation "battLoa = 360 mm"
equation "battWoa = 157 mm"
equation "battHoa = 80 mm"
equation "d14 = battWoa + 2 mm"
equation "d15 = battLoa + 2 mm"
equation "d19 = battLoa"
equation "d20 = battWoa"
equation "d21 = battHoa"
equation "cornerSize = 16 mm"
equation "d74 = cornerSize - wallThickness"
equation "d75 = cornerSize - wallThickness"
equation "gasketWidth = 2.7 mm"
equation "d99 = -( wallThickness - gasketWidth ) / 2"
equation "d113 = hoa - wallThickness"
equation "d118 = wallThickness"
equation "d119 = hoa - wallThickness"
equation "d128 = wallThickness"
equation "d130 = -gasketWidth / 2"
equation "d138 = wallThickness"
equation "d141 = wallThickness"
named bodies: "Box Base", "Battery", "Controller", "Box Back", "Box Front", "Box Left", "Box Right", "Rim", "Lid"
